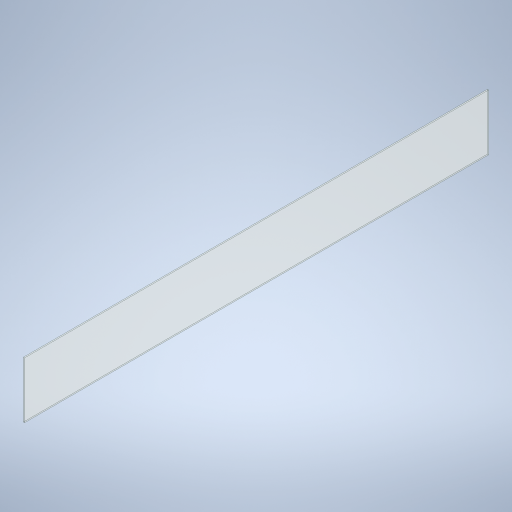
# Autodesk Inventor part: Knee_Wall
Saved by Autodesk Inventor 2024 (Build 280153000, 153)
## iProperties
Created: 2023-05-20
Part Number: Knee_Wall
Material: Concrete
Document SubType Name: Modeling
Designer: Tom
Density: 2.40731 g/cm^3
Appearance: Clear
Author: Tom
Autodesk Inventor part; units mm, degrees
ref_plane "YZ Plane" through (0, 0, 0) normal (1, 0, 0) x (0, 1, 0)
ref_plane "XZ Plane" through (0, 0, 0) normal (0, 1, 0) x (-1, 0, 0)
ref_plane "XY Plane" through (0, 0, 0) normal (0, 0, 1) x (1, 0, 0)
sketch "Sketch1" plane through (0, 0, 0) normal (1, 0, 0) x (0, 1, 0)
  line L0 (0, 0) -> (895.35, 0)
  line L1 (895.35, 0) -> (895.35, -7404.1)
  line L2 (895.35, -7404.1) -> (0, -7404.1)
  line L3 (0, -7404.1) -> (0, 0)
  dimension "d2" = 895.35
  dimension "d3" = 7404.1
  constraints: 8 end point, 2 parallel, 1 horizontal, 1 perpendicular
  measures "d2" distance of L0.start L0.end
  measures "d3" distance of L2.end L0.start
extrude "Extrusion1" add sketch "Sketch1" along normal blind 19.05
body "Solid1"
